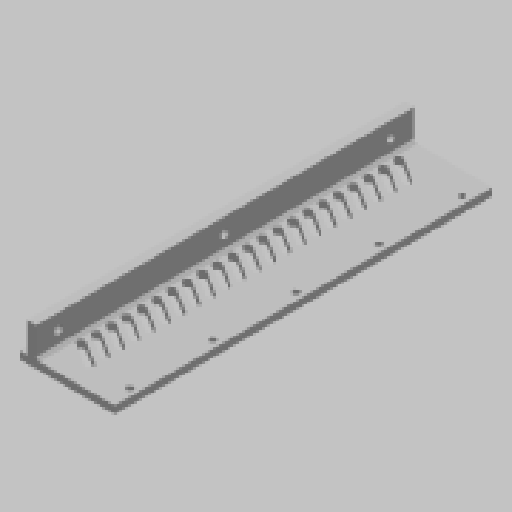
# Autodesk Inventor part: podstawa_sciana_bok
Saved by Autodesk Inventor 2024.3 (Build 283343000, 343)
## iProperties
Created: 2025-10-10
Part Number: podstawa_sciana_bok
Material: Ogólny
Document SubType Name: Modeling
Designer: User
Density: 1 g/cm^3
Appearance: Domyślna
Mass: 108.459 g
Surface Area: 449.421 cm^2
Volume: 108.459 cm^3
Author: User
Autodesk Inventor part; units mm, degrees
ref_plane "YZ Plane" through (0, 0, 0) normal (1, 0, 0) x (0, 1, 0)
ref_plane "XZ Plane" through (0, 0, 0) normal (0, 1, 0) x (-1, 0, 0)
sketch "Szkic1" plane through (0, 0, 0) normal (0, 1, 0) x (-1, 0, 0)
  line L0 (-35, 125) -> (35, 125)
  line L1 (35, 125) -> (35, -125)
  line L2 (35, -125) -> (-35, -125)
  line L3 (-35, -125) -> (-35, 125)
  line L4 (-35, 125) -> (35, -125) construction
  line L5 (35, 125) -> (-35, -125) construction
  point P0 (0, 0)
  dimension "d0" = 70
  dimension "d1" = 250
  constraints: 12 end point, 2 midpoint, 2 parallel, 1 horizontal, 1 perpendicular
  measures "d0" distance of L1.end L2.end
  measures "d1" distance of L0.end L1.end
extrude "Wyciągnięcie proste1" add sketch "Szkic1" along normal mid plane 5
sketch "Szkic2" plane through (0, 2.5, 0) normal (0, 1, 0) x (1, 0, 0)
  line L0 (-35, -125) -> (35, -125) projected
  line L1 (35, -125) -> (25, -125)
  line L2 (30, -125) -> (30, -110)
  circle A0 centre (30, -110) radius 2.15
  circle A1 centre (30, -55) radius 2.15
  circle A2 centre (30, 0) radius 2.15
  circle A3 centre (30, 55) radius 2.15
  circle A4 centre (30, 110) radius 2.15
  point P0 (0, 0)
  dimension "d4" = 10
  dimension "d5" = 15
  dimension "d6" = 4.3
  dimension "d9" = 55
  constraints: 5 centre point, 4 end point, 2 vertical, 1 coincident, 1 midpoint, 1 point on line, 8 other
  measures "d4" distance of L0.end L1.end
  measures "d5" distance of L2.start L2.end
  measures "d6" diameter of A0
  measures "d9" distance of A0.centre A1.centre
extrude "Wyciągnięcie proste2" cut sketch "Szkic2" against normal blind 16
move faces "Przesuń1" translate (7, 0, 0) faces at (-35, 0.8333, 41.6667)
ref_plane "Płaszczyzna konstrukcyjna1" through (-23, 2.5, -125) normal (-1, 0, 0) x (0, 0, 1)
sketch "Szkic3" plane through (-23, 2.5, -125) normal (-1, 0, 0) x (0, 0, 1)
  line L0 (0, 0) -> (250, 0) projected
  line L1 (0, 0) -> (0, 10)
  line L2 (0, 10) -> (15, 10)
  circle A0 centre (15, 10) radius 2.75
  circle A1 centre (70, 10) radius 2.75
  circle A2 centre (125, 10) radius 2.75
  circle A3 centre (180, 10) radius 2.75
  circle A4 centre (235, 10) radius 2.75
  line L3 (0, 0) -> (250, 0)
  line L4 (250, 0) -> (250, 20)
  line L5 (250, 20) -> (0, 20)
  line L6 (0, 20) -> (0, 0)
  point P0 (125, -2.5)
  dimension "d20" = 10
  dimension "d21" = 15
  dimension "d22" = 5.5
  dimension "d25" = 55
  dimension "d30" = 20
  constraints: 12 end point, 5 centre point, 3 horizontal, 2 parallel, 1 coincident, 1 perpendicular, 1 vertical, 8 other
  measures "d20" distance of L0.start L1.end
  measures "d21" distance of L1.end L2.end
  measures "d22" diameter of A0
  measures "d25" distance of A0.centre A1.centre
  measures "d30" distance of L4.end L3.end
extrude "Wyciągnięcie proste3" add sketch "Szkic3" against normal blind 6 contours L1 L6 L5 L4 L0 | A1 | A3
chamfer "Faza1" distance 2 angle 45 1 edges at (-17, 2.5, 0)
sketch "Szkic4" plane through (0, -2.5, 0) normal (0, -1, 0) x (1, 0, 0)
  line L0 (35, -125) -> (-15, -125) projected
  line L1 (35, -125) -> (-28, -125)
  line L2 (3.5, -125) -> (3.5, -100)
  line L3 (-28, -125) -> (3.5, -125)
  line L4 (-12.25, -125) -> (-12.25, -110)
  line L5 (-12.25, -110) -> (3.5, -100) construction
  line L6 (-10.91, -112.1105) -> (4.84, -102.1105)
  line L7 (2.16, -97.8895) -> (-13.59, -107.8895)
  arc A0 (-13.59, -107.8895) -> (-10.91, -112.1105) centre (-12.25, -110) ccw
  arc A1 (4.84, -102.1105) -> (2.16, -97.8895) centre (3.5, -100) ccw
  line L8 (-10.91, -102.1105) -> (4.84, -92.1105)
  arc A2 (-13.59, -97.8895) -> (-10.91, -102.1105) centre (-12.25, -100) ccw
  line L9 (2.16, -87.8895) -> (-13.59, -97.8895)
  arc A3 (4.84, -92.1105) -> (2.16, -87.8895) centre (3.5, -90) ccw
  line L10 (-10.91, -92.1105) -> (4.84, -82.1105)
  arc A4 (-13.59, -87.8895) -> (-10.91, -92.1105) centre (-12.25, -90) ccw
  line L11 (2.16, -77.8895) -> (-13.59, -87.8895)
  arc A5 (4.84, -82.1105) -> (2.16, -77.8895) centre (3.5, -80) ccw
  line L12 (-10.91, -82.1105) -> (4.84, -72.1105)
  arc A6 (-13.59, -77.8895) -> (-10.91, -82.1105) centre (-12.25, -80) ccw
  line L13 (2.16, -67.8895) -> (-13.59, -77.8895)
  arc A7 (4.84, -72.1105) -> (2.16, -67.8895) centre (3.5, -70) ccw
  line L14 (-10.91, -72.1105) -> (4.84, -62.1105)
  arc A8 (-13.59, -67.8895) -> (-10.91, -72.1105) centre (-12.25, -70) ccw
  line L15 (2.16, -57.8895) -> (-13.59, -67.8895)
  arc A9 (4.84, -62.1105) -> (2.16, -57.8895) centre (3.5, -60) ccw
  line L16 (-10.91, -62.1105) -> (4.84, -52.1105)
  arc A10 (-13.59, -57.8895) -> (-10.91, -62.1105) centre (-12.25, -60) ccw
  line L17 (2.16, -47.8895) -> (-13.59, -57.8895)
  arc A11 (4.84, -52.1105) -> (2.16, -47.8895) centre (3.5, -50) ccw
  line L18 (-10.91, -52.1105) -> (4.84, -42.1105)
  arc A12 (-13.59, -47.8895) -> (-10.91, -52.1105) centre (-12.25, -50) ccw
  line L19 (2.16, -37.8895) -> (-13.59, -47.8895)
  arc A13 (4.84, -42.1105) -> (2.16, -37.8895) centre (3.5, -40) ccw
  line L20 (-10.91, -42.1105) -> (4.84, -32.1105)
  arc A14 (-13.59, -37.8895) -> (-10.91, -42.1105) centre (-12.25, -40) ccw
  line L21 (2.16, -27.8895) -> (-13.59, -37.8895)
  arc A15 (4.84, -32.1105) -> (2.16, -27.8895) centre (3.5, -30) ccw
  line L22 (-10.91, -32.1105) -> (4.84, -22.1105)
  arc A16 (-13.59, -27.8895) -> (-10.91, -32.1105) centre (-12.25, -30) ccw
  line L23 (2.16, -17.8895) -> (-13.59, -27.8895)
  arc A17 (4.84, -22.1105) -> (2.16, -17.8895) centre (3.5, -20) ccw
  line L24 (-10.91, -22.1105) -> (4.84, -12.1105)
  arc A18 (-13.59, -17.8895) -> (-10.91, -22.1105) centre (-12.25, -20) ccw
  line L25 (2.16, -7.8895) -> (-13.59, -17.8895)
  arc A19 (4.84, -12.1105) -> (2.16, -7.8895) centre (3.5, -10) ccw
  line L26 (-10.91, -12.1105) -> (4.84, -2.1105)
  arc A20 (-13.59, -7.8895) -> (-10.91, -12.1105) centre (-12.25, -10) ccw
  line L27 (2.16, 2.1105) -> (-13.59, -7.8895)
  arc A21 (4.84, -2.1105) -> (2.16, 2.1105) centre (3.5, 0) ccw
  line L28 (-10.91, -2.1105) -> (4.84, 7.8895)
  arc A22 (-13.59, 2.1105) -> (-10.91, -2.1105) centre (-12.25, 0) ccw
  line L29 (2.16, 12.1105) -> (-13.59, 2.1105)
  arc A23 (4.84, 7.8895) -> (2.16, 12.1105) centre (3.5, 10) ccw
  line L30 (-10.91, 7.8895) -> (4.84, 17.8895)
  arc A24 (-13.59, 12.1105) -> (-10.91, 7.8895) centre (-12.25, 10) ccw
  line L31 (2.16, 22.1105) -> (-13.59, 12.1105)
  arc A25 (4.84, 17.8895) -> (2.16, 22.1105) centre (3.5, 20) ccw
  line L32 (-10.91, 17.8895) -> (4.84, 27.8895)
  arc A26 (-13.59, 22.1105) -> (-10.91, 17.8895) centre (-12.25, 20) ccw
  line L33 (2.16, 32.1105) -> (-13.59, 22.1105)
  arc A27 (4.84, 27.8895) -> (2.16, 32.1105) centre (3.5, 30) ccw
  line L34 (-10.91, 27.8895) -> (4.84, 37.8895)
  arc A28 (-13.59, 32.1105) -> (-10.91, 27.8895) centre (-12.25, 30) ccw
  line L35 (2.16, 42.1105) -> (-13.59, 32.1105)
  arc A29 (4.84, 37.8895) -> (2.16, 42.1105) centre (3.5, 40) ccw
  line L36 (-10.91, 37.8895) -> (4.84, 47.8895)
  arc A30 (-13.59, 42.1105) -> (-10.91, 37.8895) centre (-12.25, 40) ccw
  line L37 (2.16, 52.1105) -> (-13.59, 42.1105)
  arc A31 (4.84, 47.8895) -> (2.16, 52.1105) centre (3.5, 50) ccw
  line L38 (-10.91, 47.8895) -> (4.84, 57.8895)
  arc A32 (-13.59, 52.1105) -> (-10.91, 47.8895) centre (-12.25, 50) ccw
  line L39 (2.16, 62.1105) -> (-13.59, 52.1105)
  arc A33 (4.84, 57.8895) -> (2.16, 62.1105) centre (3.5, 60) ccw
  line L40 (-10.91, 57.8895) -> (4.84, 67.8895)
  arc A34 (-13.59, 62.1105) -> (-10.91, 57.8895) centre (-12.25, 60) ccw
  line L41 (2.16, 72.1105) -> (-13.59, 62.1105)
  arc A35 (4.84, 67.8895) -> (2.16, 72.1105) centre (3.5, 70) ccw
  line L42 (-10.91, 67.8895) -> (4.84, 77.8895)
  arc A36 (-13.59, 72.1105) -> (-10.91, 67.8895) centre (-12.25, 70) ccw
  line L43 (2.16, 82.1105) -> (-13.59, 72.1105)
  arc A37 (4.84, 77.8895) -> (2.16, 82.1105) centre (3.5, 80) ccw
  line L44 (-10.91, 77.8895) -> (4.84, 87.8895)
  arc A38 (-13.59, 82.1105) -> (-10.91, 77.8895) centre (-12.25, 80) ccw
  line L45 (2.16, 92.1105) -> (-13.59, 82.1105)
  arc A39 (4.84, 87.8895) -> (2.16, 92.1105) centre (3.5, 90) ccw
  line L46 (-10.91, 87.8895) -> (4.84, 97.8895)
  arc A40 (-13.59, 92.1105) -> (-10.91, 87.8895) centre (-12.25, 90) ccw
  line L47 (2.16, 102.1105) -> (-13.59, 92.1105)
  arc A41 (4.84, 97.8895) -> (2.16, 102.1105) centre (3.5, 100) ccw
  line L48 (-10.91, 97.8895) -> (4.84, 107.8895)
  arc A42 (-13.59, 102.1105) -> (-10.91, 97.8895) centre (-12.25, 100) ccw
  line L49 (2.16, 112.1105) -> (-13.59, 102.1105)
  arc A43 (4.84, 107.8895) -> (2.16, 112.1105) centre (3.5, 110) ccw
  point P0 (0, 0)
  point P1 (-4.375, -105)
  point P2 (-12.25, -112.5)
  point P3 (3.5, -102.9613)
  dimension "d36" = 25
  dimension "d37" = 5
  dimension "d40" = 10
  constraints: 100 end point, 88 point on circle, 44 centre point, 4 tangent, 3 midpoint, 3 vertical, 1 horizontal, 1 parallel, 210 other
  measures "d36" distance of L2.start L2.end
  measures "d37" diameter of A1
  measures "d40" distance of L6.start L8.start
extrude "Wyciągnięcie proste4" cut sketch "Szkic4" against normal blind 10 contours L6 A0 L7 A1 | A2 L9 A3 L8 | A4 L11 A5 L10 | A6 L13 A7 L12 | A8 L15 A9 L14 | A10 L17 A11 L16 | A12 L19 A13 L18 | A14 L21 A15 L20 | A16 L23 A17 L22 | A18 L25 A19 L24 | A20 L27 A21 L26 | A22 L29 A23 L28 | A24 L31 A25 L30 | A26 L33 A27 L32 | A28 L35 A29 L34 | A30 L37 A31 L36 | A32 L39 A33 L38 | A34 L41 A35 L40 | A36 L43 A37 L42 | A38 L45 A39 L44 | A40 L47 A41 L46 | A42 L49 A43 L48
